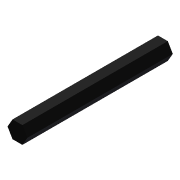
# Autodesk Inventor part: Axle
Saved by Autodesk Inventor 2011 (Build 150239000, 239)
## iProperties
Created: 2014-09-14
Part Number: Axle
Document SubType Name: Modeling
Designer: Family Room
Density: 1 g/cm^3
Author: Family Room
Autodesk Inventor part; units mm, degrees
ref_plane "YZ Plane" through (0, 0, 0) normal (1, 0, 0) x (0, 1, 0)
ref_plane "XZ Plane" through (0, 0, 0) normal (0, 1, 0) x (-1, 0, 0)
ref_plane "XY Plane" through (0, 0, 0) normal (0, 0, 1) x (1, 0, 0)
sketch "Sketch1" plane through (0, 0, 0) normal (0, 0, 1) x (1, 0, 0)
  line L0 (3.6662, 6.35) -> (7.3323, 0)
  line L1 (7.3323, 0) -> (3.6662, -6.35)
  line L2 (3.6662, -6.35) -> (-3.6662, -6.35)
  line L3 (-3.6662, -6.35) -> (-7.3323, 0)
  line L4 (-7.3323, 0) -> (-3.6662, 6.35)
  line L5 (-3.6662, 6.35) -> (3.6662, 6.35)
  point P0 (0, 0)
  point P1 (0, 0)
  point P2 (0, 6.35)
  constraints: 12 end point, 1 midpoint, 13 other
extrude "Extrusion1" add sketch "Sketch1" along normal blind 107.95
sketch "Sketch2" plane through (0, 0, 107.95) normal (0, 0, 1) x (1, 0, 0)
  line L0 (7.3323, 0) -> (3.6662, -6.35) projected
  line L1 (3.6662, 6.35) -> (7.3323, 0) projected
  line L2 (-3.6662, 6.35) -> (3.6662, 6.35) projected
  line L3 (-7.3323, 0) -> (-3.6662, 6.35) projected
  line L4 (-3.6662, -6.35) -> (-7.3323, 0) projected
  line L5 (3.6662, -6.35) -> (-3.6662, -6.35) projected
  circle A0 centre (0, 0) radius 7.3323
  constraints: 1 coincident, 3 other
sketch "Sketch3" plane through (0, 0, 0) normal (0, 0, -1) x (-1, 0, 0)
  line L0 (-3.6662, 6.35) -> (-7.3323, 0) projected
  line L1 (-7.3323, 0) -> (-3.6662, -6.35) projected
  line L2 (-3.6662, -6.35) -> (3.6662, -6.35) projected
  line L3 (3.6662, -6.35) -> (7.3323, 0) projected
  line L4 (7.3323, 0) -> (3.6662, 6.35) projected
  line L5 (3.6662, 6.35) -> (-3.6662, 6.35) projected
  circle A0 centre (0, 0) radius 7.3323
  constraints: 1 coincident, 3 other
body "Solid1"
